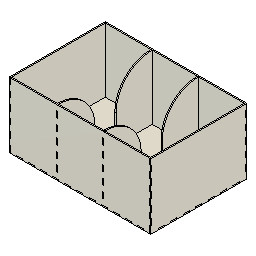
model (Autodesk Fusion 360 design; units mm, degrees)
Autodesk Fusion 360 part; units mm, degrees
sketch "Inner" plane through (0, 0, 0) normal (1, 0, 0) x (0, 0, -1) in component "Main"
  line L0 (-50.8, 0) -> (-50.8, 133.35)
  arc A0 (-50.8, 133.35) -> (-222.25, 304.8) centre (-222.25, 133.35) ccw
  line L1 (-222.25, 304.8) -> (-222.25, 0)
  line L2 (-50.8, 0) -> (0, 0)
  line L3 (-50.8, 0) -> (-222.25, 0)
  line L4 (-222.25, 55.4182) -> (-228.15, 55.4182)
  line L5 (-228.15, 55.4182) -> (-228.15, 27.7091)
  line L6 (-228.15, 27.7091) -> (-222.25, 27.7091)
  line L7 (-197.7571, 0) -> (-197.7571, -5.9)
  line L8 (-197.7571, -5.9) -> (-173.2643, -5.9)
  line L9 (-173.2643, -5.9) -> (-173.2643, 0)
  line L10 (-222.25, 304.8) -> (222.25, 304.8)
  line L11 (222.25, 304.8) -> (222.25, 0)
  line L12 (222.25, 0) -> (0, 0)
  dimension "d64" = 27.7091
  dimension "d76" = 24.4929
  dimension "d77" = 24.4929
  dimension "d87" = 27.7091
  dimension "d88" = 5.9
  dimension "d89" = 222.25
  dimension "d90" = 50.8
  dimension "d91" = 304.8
  dimension "d92" = 444.5
  constraint vertical L1
  constraint coincident A0.centre L1
  constraint tangent L0 A0
  constraint coincident L2.end L12.end
  constraint perpendicular L0 L2
  constraint perpendicular L1 L3
  constraint perpendicular L0 L3
  constraint coincident L1 L4.start
  constraint perpendicular L1 L4
  constraint perpendicular L4 L5
  constraint coincident L1 L6.end
  constraint perpendicular L1 L6
  constraint coincident L3 L7.start
  constraint perpendicular L3 L7
  constraint perpendicular L7 L8
  constraint coincident L3 L9.end
  constraint perpendicular L3 L9
  constraint equal L6 L7
  constraint perpendicular L1 L10
  constraint perpendicular L10 L11
  constraint perpendicular L11 L12
  constraint coincident A0.end L1.start
  measures "d64" distance of L1.end L6
  measures "d76" distance of L7.end L8.end
  measures "d77" distance of L1.end L7
  measures "d87" distance of L4.end L5.end
  measures "d88" distance of L5.end L6.end
  measures "d89" distance of L2.end L1.end
  measures "d90" distance of L0.start L2.end
  measures "d91" distance of A0.end L1.end
  measures "d92" distance of A0.end L10.end
extrude "Extrude5" add sketch "Inner" along normal mid plane 5.9 from surface at -110.0667 contours L0 A0 L1 L3 makes body 1 in component "Main"
extrude "Extrude10" add sketch "Inner" along normal blind 5.9 from surface at -113.0167 contours L1 L4 L5 L6 bodies 1 in component "Main"
extrude "Extrude11" add sketch "Inner" along normal blind 5.9 from surface at -113.0167 contours L3 L7 L8 L9 bodies 1 in component "Main"
pattern_linear "R-Pattern5" count 3 spacing 48.9857 along (0, 0, -1) of "Extrude11" in component "Main"
pattern_linear "R-Pattern4" count 5 spacing 55.4182 along (0, 1, 0) of "Extrude10" in component "Main"
mirror "Mirror4" about plane through (0, 0, 0) normal (0, 0, 1) of bodies 1 makes body 2 in component "Main"
extrude "Extrude12" add sketch "Inner" along normal blind 5.9 from surface at -107.1167 separate body contours L0 A0 L1 L3 | L0 A0 L2 L10 L11 L12 makes body 3 in component "Main"
fillet "Fillet1" radius 5 4 edges at (-104.1667, 304.8, 222.25) (-104.1667, 304.8, -222.25) (-104.1667, 0, -222.25) (-104.1667, 0, 222.25) on bodies 3 in component "Main"
mirror "Mirror3" about plane through (0, 0, 0) normal (1, 0, 0) of bodies 1 2 3 makes body 4 at (113.0167, 72.1591, 132.4429) makes body 5 at (113.0167, 72.1591, -132.4429) makes body 6 at (101.2167, 203.2, 72.4167) in component "Main"
sketch "Floor" plane through (0, 0, 0) normal (0, 1, 0) x (1, 0, 0) in component "Main"
  line L0 (-336.1, 228.15) -> (336.1, 228.15)
  line L1 (336.1, 228.15) -> (336.1, -228.15)
  line L2 (336.1, -228.15) -> (-336.1, -228.15)
  line L3 (-336.1, -228.15) -> (-336.1, 228.15)
  line L4 (-330.2, 222.25) -> (330.2, 222.25)
  line L5 (330.2, 222.25) -> (330.2, -222.25)
  line L6 (330.2, -222.25) -> (-330.2, -222.25)
  line L7 (-330.2, -222.25) -> (-330.2, 222.25)
  line L8 (-330.2, 222.25) -> (330.2, -222.25) construction
  line L9 (-330.2, 222.25) -> (-336.1, 222.25)
  line L10 (-330.2, 222.25) -> (-330.2, 228.15)
  line L11 (330.2, -222.25) -> (336.1, -222.25)
  line L12 (330.2, -222.25) -> (330.2, -228.15)
  line L13 (330.2, 222.25) -> (330.2, 228.15)
  line L14 (330.2, 222.25) -> (336.1, 222.25)
  line L15 (-330.2, -222.25) -> (-336.1, -222.25)
  line L16 (-330.2, -222.25) -> (-330.2, -228.15)
  line L17 (107.1167, -222.25) -> (107.1167, -228.15)
  line L18 (113.0167, -222.25) -> (113.0167, -228.15)
  line L19 (107.1167, 222.25) -> (107.1167, 228.15)
  line L20 (113.0167, 222.25) -> (113.0167, 228.15)
  line L21 (107.1167, 225.2) -> (113.0167, 225.2) construction
  line L22 (107.1167, -225.2) -> (113.0167, -225.2) construction
  line L23 (110.0667, -225.2) -> (110.0667, 225.2) construction
  line L24 (-110.0667, 225.2) -> (-110.0667, -225.2) construction
  line L25 (-113.0167, 225.2) -> (-107.1167, 225.2) construction
  line L26 (-113.0167, 222.25) -> (-113.0167, 228.15)
  line L27 (-107.1167, 222.25) -> (-107.1167, 228.15)
  line L28 (-113.0167, -222.25) -> (-113.0167, -228.15)
  line L29 (-107.1167, -222.25) -> (-107.1167, -228.15)
  line L30 (-113.0167, -225.2) -> (-107.1167, -225.2) construction
  line L31 (-330.2, 0) -> (-110.0667, 0) construction
  line L32 (-110.0667, 0) -> (110.0667, 0) construction
  line L33 (110.0667, 0) -> (330.2, 0) construction
  line L34 (-336.1, 192.6167) -> (-330.2, 192.6167)
  line L35 (-301.487, 228.15) -> (-301.487, 222.25)
  line L36 (-333.15, 222.25) -> (-333.15, 192.6167) construction
  line L37 (-330.2, 225.2) -> (-301.487, 225.2) construction
  line L38 (-301.487, -222.25) -> (-301.487, -228.15)
  line L39 (330.2, 192.6167) -> (336.1, 192.6167)
  line L40 (333.15, 192.6167) -> (333.15, 222.25) construction
  line L41 (-330.2, -225.2) -> (-301.487, -225.2) construction
  dimension "d1" = 444.5
  dimension "d2" = 660.4
  dimension "d6" = 5.9
  dimension "d30" = 28.713
  dimension "d31" = 29.6333
  constraint horizontal L0
  constraint vertical L1
  constraint horizontal L2
  constraint vertical L3
  constraint horizontal L4
  constraint vertical L5
  constraint horizontal L6
  constraint vertical L7
  constraint midpoint origin L8
  constraint coincident L3 L9.end
  constraint perpendicular L3 L9
  constraint coincident L0 L10.end
  constraint perpendicular L0 L10
  constraint coincident L1 L11.end
  constraint perpendicular L1 L11
  constraint coincident L2 L12.end
  constraint perpendicular L2 L12
  constraint equal L11 L12
  constraint equal L10 L11
  constraint equal L9 L10
  constraint coincident L0 L13.end
  constraint perpendicular L0 L13
  constraint coincident L1 L14.end
  constraint perpendicular L1 L14
  constraint coincident L3 L15.end
  constraint perpendicular L3 L15
  constraint coincident L2 L16.end
  constraint perpendicular L2 L16
  constraint coincident L4 L20.start
  constraint coincident L6 L18.start
  constraint coincident L4 L19.start
  constraint coincident L6 L17.start
  constraint coincident L2 L17.end
  constraint perpendicular L2 L17
  constraint coincident L2 L18.end
  constraint perpendicular L2 L18
  constraint coincident L0 L19.end
  constraint perpendicular L0 L19
  constraint coincident L0 L20.end
  constraint perpendicular L0 L20
  constraint midpoint L19 L21.start
  constraint midpoint L20 L21.end
  constraint midpoint L17 L22.start
  constraint midpoint L18 L22.end
  constraint midpoint L22 L23.start
  constraint midpoint L21 L23.end
  constraint perpendicular L21 L23
  constraint equal L21 L22
  constraint equal L10 L22
  constraint perpendicular L6 L24
  constraint perpendicular L24 L25
  constraint midpoint L24.start L25
  constraint coincident L4 L26.start
  constraint coincident L0 L26.end
  constraint perpendicular L0 L26
  constraint coincident L4 L27.start
  constraint coincident L0 L27.end
  constraint perpendicular L0 L27
  constraint midpoint L25.end L27
  constraint midpoint L25.start L26
  constraint coincident L6 L28.start
  constraint coincident L2 L28.end
  constraint perpendicular L2 L28
  constraint coincident L6 L29.start
  constraint coincident L2 L29.end
  constraint perpendicular L2 L29
  constraint midpoint L28 L30.start
  constraint midpoint L29 L30.end
  constraint midpoint L24.end L30
  constraint midpoint L7 L31.start
  constraint midpoint L24 L31.end
  constraint midpoint L23 L32.end
  constraint perpendicular L23 L32
  constraint midpoint L5 L33.end
  constraint perpendicular L5 L33
  constraint equal L32 L33
  constraint equal L31 L32
  constraint equal L25 L30
  constraint equal L10 L25
  constraint coincident L3 L34.start
  constraint coincident L7 L34.end
  constraint perpendicular L7 L34
  constraint coincident L0 L35.start
  constraint coincident L4 L35.end
  constraint perpendicular L4 L35
  constraint midpoint L9 L36.start
  constraint midpoint L34 L36.end
  constraint midpoint L10 L37.start
  constraint midpoint L35 L37.end
  constraint coincident L6 L38.start
  constraint coincident L2 L38.end
  constraint perpendicular L2 L38
  constraint coincident L5 L39.start
  constraint coincident L1 L39.end
  constraint perpendicular L1 L39
  constraint midpoint L39 L40.start
  constraint midpoint L14 L40.end
  constraint midpoint L16 L41.start
  constraint midpoint L38 L41.end
  constraint equal L37 L41
  constraint equal L36 L40
  measures "d1" distance of L4.end L5.end
  measures "d2" distance of L4.start L4.end
  measures "d6" distance of L4.start L10.end
  measures "d30" distance of L37.start L37.end
  measures "d31" distance of L36.start L36.end
extrude "Extrude1" add sketch "Floor" against normal blind 5.9 separate body contours L0 L4 L10 L35 | L3 L7 L9 L34 | L0 L4 L26 L35 | L4 L5 L6 L7 | L3 L7 L15 L34 | L0 L4 L26 L27 | L0 L4 L19 L27 | L2 L6 L16 L38 | L0 L4 L19 L20 | L2 L6 L28 L38 | L0 L4 L13 L20 | L2 L6 L28 L29 | L2 L6 L17 L29 | L1 L5 L14 L39 | L2 L6 L17 L18 | L1 L5 L11 L39 | L2 L6 L12 L18 makes body 7 in component "Main"
extrude "Extrude6" cut sketch "Floor" against normal blind 5.9 contours L0 L4 L10 L35 | L2 L6 L16 L38 bodies 7 in component "Main"
pattern_linear "R-Pattern1" count 12 spacing 57.4261 along (1, 0, 0) of "Extrude6" in component "Main"
extrude "Extrude7" cut sketch "Floor" against normal blind 5.9 contours L3 L7 L9 L34 | L1 L5 L14 L39 bodies 7 in component "Main"
pattern_linear "R-Pattern2" count 8 spacing 59.2667 along (0, 0, 1) of "Extrude7" in component "Main"
combine "Combine3" operation cut target body 7 tool bodies 1 2 4 5 keep tools in component "Main"
extrude "Extrude2" add sketch "Floor" along normal blind 304.8 and the other way blind 5.9 separate body contours L3 L7 L9 L34 | L3 L7 L15 L34 makes body 8 in component "Main"
extrude "Extrude8" add sketch "Floor" along normal blind 27.7091 contours L0 L3 L9 L10 | L2 L3 L15 L16 bodies 8 in component "Main"
pattern_linear "R-Pattern3" count 6 spacing 55.4182 along (0, 1, 0) of "Extrude8" in component "Main"
extrude "Extrude9" add sketch "Floor" against normal blind 5.9 contours L0 L3 L9 L10 | L2 L3 L15 L16 bodies 8 in component "Main"
combine "Combine1" operation cut target body 8 tool bodies 7 keep tools in component "Main"
mirror "Mirror1" about plane through (0, 0, 0) normal (1, 0, 0) of bodies 8 makes body 9 in component "Main"
extrude "Extrude3" add sketch "Floor" along normal blind 304.8 and the other way blind 5.9 separate body contours L0 L3 L9 L10 | L0 L4 L10 L35 | L0 L4 L26 L35 | L0 L4 L26 L27 | L0 L4 L19 L27 | L0 L4 L19 L20 | L0 L4 L13 L20 | L0 L1 L13 L14 makes body 10 in component "Main"
combine "Combine2" operation cut target body 10 tool bodies 8 9 7 2 1 4 5 keep tools in component "Main"
mirror "Mirror2" about plane through (0, 0, 0) normal (0, 0, 1) of bodies 10 makes body 11 in component "Main"
component "Main" placed x (1, 0, 0) y (0, 1, 0) z (0, 0, 1) at (0, 0, 0)
hidden bodies 3 6
equation "d1 = Width"
equation "d2 = Length"
equation "d6 = Thick"
equation "d7 = -Thick"
equation "d9 = Height"
equation "d11 = Height"
equation "d16 = ( -Length / 6 )"
equation "d17 = Thick"
equation "Length = 26 in"
equation "Width = 17.5 in"
equation "Thick = 5.9 mm"
equation "Height = 12 in"
equation "DoorW = 4 in"
equation "LengthCount = 12"
equation "LengthTab = Length / ( 2 * LengthCount - 1 )"
equation "WidthCount = 8"
equation "WidthTab = Width / ( 2 * WidthCount - 1 )"
equation "HeightCount = 6"
equation "HeightTab = Height / ( 2 * HeightCount - 1 )"
equation "d30 = LengthTab"
equation "d31 = WidthTab"
equation "d32 = -Thick"
equation "d34 = LengthCount"
equation "d36 = 2 * LengthTab"
equation "d38 = -Thick"
equation "d40 = WidthCount"
equation "d42 = 2 * WidthTab"
equation "d44 = Thick"
equation "d46 = Thick"
equation "d48 = HeightTab"
equation "d50 = HeightCount"
equation "d52 = -2 * HeightTab"
equation "d54 = -Thick"
equation "d64 = HeightTab"
equation "d65 = -( Length / 6 + Thick / 2 )"
equation "d66 = Thick"
equation "d68 = HeightCount - 1"
equation "d70 = -2 * HeightTab"
equation "InnerCount = 4"
equation "InnerTab = ( Width - DoorW ) / 2 / ( 2 * InnerCount - 1 )"
equation "d76 = InnerTab"
equation "d77 = InnerTab"
equation "d78 = -Length / 6 - Thick / 2"
equation "d79 = Thick"
equation "d81 = InnerCount - 1"
equation "d83 = -2 * InnerTab"
equation "d87 = HeightTab"
equation "d88 = Thick"
equation "d89 = Width / 2"
equation "d90 = DoorW / 2"
equation "d91 = Height"
equation "d92 = Width"
equation "d96 = -Length / 6 + Thick / 2"
equation "d97 = Thick"
named bodies: "Bottom", "Left", "Back", "InnerLF", "Right", "Front", "InnerRF", "InnerLB", "InnerRB", "RemovableL", "RemovableR"
